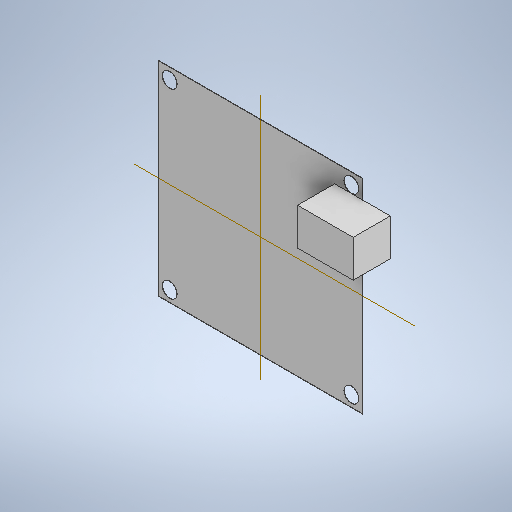
# Autodesk Inventor part: 모터드라이버
Saved by Autodesk Inventor 2025 (Build 290162000, 162)
## iProperties
Created: 2024-06-01
Part Number: 모터드라이버
Material: 일반
Document SubType Name: Modeling
Designer: ckhye
Density: 1 g/cm^3
Appearance: 기본값
Author: ckhye
Autodesk Inventor part; units mm, degrees
ref_plane "YZ Plane" through (0, 0, 0) normal (1, 0, 0) x (0, 1, 0)
ref_plane "XZ Plane" through (0, 0, 0) normal (0, 1, 0) x (-1, 0, 0)
ref_plane "XY Plane" through (0, 0, 0) normal (0, 0, 1) x (1, 0, 0)
sketch "스케치2" plane through (0, 0, 0) normal (0, 0, 1) x (1, 0, 0)
  line L0 (-27.5, 27.5) -> (27.5, 27.5)
  line L1 (27.5, 27.5) -> (27.5, -27.5)
  line L2 (27.5, -27.5) -> (-27.5, -27.5)
  line L3 (-27.5, -27.5) -> (-27.5, 27.5)
  line L4 (-27.5, 27.5) -> (27.5, -27.5) construction
  line L5 (27.5, 27.5) -> (-27.5, -27.5) construction
  point P0 (0, 0)
  dimension "d0" = 55
  dimension "d1" = 55
  constraints: 12 end point, 2 midpoint, 2 parallel, 1 horizontal, 1 perpendicular
  measures "d0" distance of L1.end L2.end
  measures "d1" distance between parallel lines of L2 L0
extrude "돌출1" add sketch "스케치2" along normal blind 0.1
sketch "스케치3" plane through (0, 0, 0.1) normal (0, 0, 1) x (1, 0, 0)
  line L0 (27.5, -27.5) -> (27.5, 27.5) projected
  line L1 (27.5, 27.5) -> (-27.5, 27.5) projected
  circle A0 centre (24.5, 24.5) radius 3
  circle A1 centre (-24.5, 24.5) radius 3
  circle A2 centre (-24.5, -24.5) radius 3
  circle A3 centre (24.5, -24.5) radius 3
  line L2 (-27.5, 27.5) -> (-27.5, -27.5) projected
  line L3 (-27.5, -27.5) -> (27.5, -27.5) projected
  circle A4 centre (24.5, 24.5) radius 2
  circle A5 centre (-24.5, 24.5) radius 2
  circle A6 centre (-24.5, -24.5) radius 2
  circle A7 centre (24.5, -24.5) radius 2
  point P0 (0, 0)
  dimension "d5" = 6
  dimension "d6" = 6
  dimension "d7" = 6
  dimension "d8" = 6
  dimension "d9" = 4
  dimension "d10" = 4
  dimension "d11" = 4
  dimension "d12" = 4
  constraints: 8 centre point, 8 tangent, 4 coincident
  measures "d5" diameter of A0
  measures "d6" diameter of A1
  measures "d7" diameter of A2
  measures "d8" diameter of A3
  measures "d9" diameter of A4
  measures "d10" diameter of A5
  measures "d11" diameter of A6
  measures "d12" diameter of A7
extrude "돌출2" cut sketch "스케치3" against normal up to surface (0.1 mm away) contours A4 | A5 | A6 | A7
sketch "스케치4" plane through (0, 0, 0.1) normal (0, 0, 1) x (1, 0, 0)
  line L0 (20, 12.5) -> (35, 12.5)
  line L1 (35, 12.5) -> (35, 22.5)
  line L2 (35, 22.5) -> (20, 22.5)
  line L3 (20, 22.5) -> (20, 12.5)
  line L4 (20, 12.5) -> (35, 22.5) construction
  line L5 (35, 12.5) -> (20, 22.5) construction
  line L6 (27.5, -27.5) -> (27.5, 27.5) projected
  circle A0 centre (24.5, 24.5) radius 2 projected
  point P0 (0, 0)
  point P1 (27.5, 17.5)
  dimension "d15" = 15
  dimension "d16" = 10
  constraints: 12 end point, 2 midpoint, 2 parallel, 1 horizontal, 1 perpendicular, 1 point on line, 1 tangent
  measures "d15" distance of L2.end L1.end
  measures "d16" distance between parallel lines of L2 L0
extrude "돌출3" add sketch "스케치4" along normal blind 10 contours L3 L2 L6 L0 | L6 L2 L1 L0
